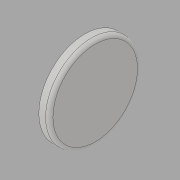
# Autodesk Inventor part: Connector_pin_collar
Saved by Autodesk Inventor 2019.3 (Build 233278000, 278)
## iProperties
Created: 2019-02-05
Part Number: Connector_pin_collar
Material: Generic
Document SubType Name: Modeling
Designer: Varga Daniel
Density: 1 g/cm^3
Appearance: Default
Author: Varga Daniel
Autodesk Inventor part; units mm, degrees
ref_plane "YZ Plane" through (0, 0, 0) normal (1, 0, 0) x (0, 1, 0)
ref_plane "XZ Plane" through (0, 0, 0) normal (0, 1, 0) x (-1, 0, 0)
ref_plane "XY Plane" through (0, 0, 0) normal (0, 0, 1) x (1, 0, 0)
derived "Connector_pin_base.ipt"
sketch "Pin_base_sketch" plane through (0, 0, 0) normal (0, 0, 1) x (1, 0, 0)
  line L0 (0, 0) -> (23.0918, 0) construction
  line L1 (0, 0) -> (0, 6.22) construction
  line L2 (0, 3.75) -> (0.55, 3.75)
  line L3 (0.85, 3.45) -> (0.85, 2.5)
  line L4 (0.85, 2.5) -> (10, 2.5)
  line L5 (10, 2.5) -> (10, 0)
  line L6 (0, 0) -> (0, 3.75)
  line L7 (0, 0) -> (10, 0)
  line L8 (9.25, 2.5) -> (9.25, 2.625)
  line L9 (10, 2.5) -> (10, 2.5024)
  arc A0 (10, 2.5024) -> (9.9256, 2.6604) centre (9.795, 2.5024) ccw
  arc A1 (9.9256, 2.6604) -> (9.25, 2.625) centre (9.6071, 2.275) ccw
  line L10 (9.9256, 2.6604) -> (9.9256, -0.0789) construction
  line L11 (8.9584, 2.775) -> (10.3858, 2.775) construction
  arc A2 (0.85, 3.45) -> (0.55, 3.75) centre (0.55, 3.45) ccw
  line L12 (0.85, 2.5) -> (0.85, 0)
  line L13 (-0.85, 2.5) -> (-0.85, 0)
  line L14 (-0.85, 3.45) -> (-0.85, 2.5)
  arc A3 (-0.55, 3.75) -> (-0.85, 3.45) centre (-0.55, 3.45) ccw
  line L15 (0, 3.75) -> (-0.55, 3.75)
  line L16 (0, 0) -> (-23.0918, 0) construction
  line L17 (0, 0) -> (-10, 0)
  line L18 (-0.85, 2.5) -> (-10, 2.5)
  line L19 (-9.25, 2.5) -> (-9.25, 2.625)
  arc A4 (-9.25, 2.625) -> (-9.9256, 2.6604) centre (-9.6071, 2.275) ccw
  arc A5 (-9.9256, 2.6604) -> (-10, 2.5024) centre (-9.795, 2.5024) ccw
  line L20 (-10, 2.5) -> (-10, 2.5024)
  line L21 (-8.9584, 2.775) -> (-10.3858, 2.775) construction
  line L22 (-9.9256, 2.6604) -> (-9.9256, -0.0789) construction
  line L23 (-10, 2.5) -> (-10, 0)
  line L24 (9.625, 3.2563) -> (9.625, -1.1868) construction
revolve "Revolution1" add sketch "Pin_base_sketch" angle 360 about axis through (0, 0, 0) along (1, 0, 0) contours L2 A2 L3 L12 L7 L6
body "Solid1"
